Autodesk Fusion 360 part; units mm, degrees
note: some values were not read from the file. Chosen so that the rebuilt part matches the saved one: which face or edge a step refers to.
(part 2 of 2)
  line L527 (-26.0359, -3.6443) -> (-26.0026, -3.5739) construction
  line L528 (-26.0026, -3.5739) -> (-25.9789, -3.5255) construction
  line L529 (-25.9789, -3.5255) -> (-25.9665, -3.5003) construction
  line L530 (-121, -21.875) -> (-119, -21.875)
  line L531 (-119, -21.875) -> (-119, -56.875)
  line L532 (-119, -56.875) -> (-121, -56.875)
  line L533 (-60.5, -78.75) -> (-60.5, 0.0063) construction
  line L534 (-2, -56.875) -> (0, -56.875)
  line L535 (-2, -21.875) -> (-2, -56.875)
  line L536 (0, -21.875) -> (-2, -21.875)
  point P0 (0, -78.75)
  dimension "d4" = 5
  dimension "PlateWidthY" = 78.75
  dimension "d8" = 11.35
  dimension "OffsetY" = 6.725
  dimension "OffsetX" = 16.19
  dimension "PlateWidthX" = 117
  dimension "d21" = 6.875
  dimension "CapHolderWidth" = 13.4
  dimension "d27" = 2
  dimension "d28" = 2
  dimension "d29" = 2
  dimension "d38" = 2
  dimension "d39" = 80
  dimension "d47" = 2
  dimension "d48" = 2.5
  dimension "CapHolderAngle" = 45
  dimension "d50" = 2
  dimension "d51" = 35
  dimension "d52" = 17.5
  dimension "d53" = 10
  constraint horizontal L45
  constraint vertical L46
  constraint horizontal L47
  constraint vertical L48
  constraint coincident L54.start L53
  constraint perpendicular L49 L54
  constraint perpendicular L49 L50
  constraint parallel L49 L52
  constraint equal L51 L53
  constraint coincident L54 L53.end
  constraint coincident L50.start L51.start
  constraint coincident L46.start L56.start
  constraint coincident L45.end L56.end
  constraint coincident L55.end A0.centre
  constraint equal L50 L54
  constraint midpoint L49 L55.start
  constraint coincident origin L48
  constraint coincident L45 origin
  constraint tangent L48 A1
  constraint tangent L45 A1
  constraint coincident P0 L47
  constraint coincident P0 L48
  constraint tangent L47 A2
  constraint tangent L48 A2
  constraint tangent L46 A3
  constraint tangent L47 A3
  constraint perpendicular L47 L58
  constraint perpendicular L57 L59
  constraint equal L57 L58
  constraint perpendicular L58 L59
  constraint coincident L47 L57.start
  constraint midpoint L48 L60.start
  constraint coincident L46 L60.end
  constraint perpendicular L46 L60
  constraint symmetric L57.start L60 L62.start
  constraint symmetric L57.end L60 L61.end
  constraint symmetric L58.start L60 L61.start
  constraint symmetric L58.end L60 L63.end
  constraint perpendicular L52 L64
  constraint perpendicular L64 L65
  constraint perpendicular L65 L66
  constraint perpendicular L49 L55
  constraint coincident L48 L67.end
  constraint perpendicular L48 L67
  constraint coincident L46 L530.start
  constraint perpendicular L46 L530
  constraint coincident L46 L532.end
  constraint perpendicular L46 L532
  constraint perpendicular L531 L532
  constraint midpoint L47 L533.start
  constraint perpendicular L45 L533
  constraint symmetric L530.start L533 L536.start
  constraint symmetric L530.end L533 L535.start
  constraint symmetric L531.end L533 L534.start
  constraint symmetric L532.end L533 L534.end
  measures "d4" distance of L49 L52
  measures "PlateWidthY" distance of origin P0
  measures "d8" diameter of A0
  measures "OffsetY" distance of L45 L55.end
  measures "OffsetX" distance of L48 L55.end
  measures "PlateWidthX" distance of L45.end origin
  measures "d21" distance of L55.start L55.end
  measures "CapHolderWidth" distance of L49.start L49.end
  measures "d27" radius of A1
  measures "d28" radius of A2
  measures "d29" radius of A3
  measures "d38" distance of L58.start L58.end
  measures "d39" distance of L57.end L58.start
  measures "d47" distance of L52.end L64.end
  measures "d48" distance of L49.start L53.end
  measures "CapHolderAngle" angle of L55 L67
  measures "d50" distance of L530.start L530.end
  measures "d51" distance of L534.start L535.start
  measures "d52" distance of L60 L532
  measures "d53" distance of L64.end L65.end
extrude "Extrude1" add sketch "Sketch1" along normal blind 10 separate body contours L0 L1 L2 L3 L4 L5 L6 L7 | S0 L8 S1 S2 S3 L9 L10 L11 L12 L13 L14 S4 S5 L15 L17 L18 L19 L20 L21 L22 L23 L24 L25 L26 L27 L28 S6 S7 S8 S9 L29 L31 L32 L33 S10 S11 S12 S13 L34 S14 S15 S16 S17 L35 S18 L36 S19 S20 S21 S22 S23 S24 S25 L37 S26 S27 S28 L38 S29 S30 L45 L46 L47 L48 L56 A1 A2 A3 L57 L58 L59 L61 L62 L63 L530 L531 L532 L534 L535 L536 | S0 L8 S1 S2 S3 L9 L10 L11 L12 L13 L14 S4 S5 L61 | S1 S2 L15 L16 L17 L26 L27 L29 L30 L31 S20 S21 L45 L61 L62 L63 | S1 S2 L61 | S18 L36 S19 S20 S21 S22 S23 S24 S25 L37 S26 S27 S28 L38 S29 S30 L61 | S20 S21 L61 | L15 L17 L18 L19 L20 L21 L22 L23 L24 L25 L61 | L15 L16 L17 L61 | L26 L27 L61 | L26 L27 L28 S6 S7 S8 S9 L61 | L46 L530 L531 L532 | L29 L31 L32 L33 S10 S11 S12 S13 L34 S14 S15 S16 S17 L35 L61 | L29 L30 L31 L61 | L48 L534 L535 L536 | L47 L57 L58 L59 | L39 L40 L41 L42 L43 L44 | L49 L50 L51 L52 L53 L54 | L52 L64 L65 L66 | A0 makes body 2
extrude "Extrude2" cut sketch "Sketch1" along normal up to surface (10 mm away) contours L49 L50 L51 L52 L53 L54 | L52 L64 L65 L66 | A0 bodies 2
pattern_linear "R-Pattern1" count 6 spacing 18 along (-1, 0, 0) count 4 spacing 18 along (0, -1, 0) of "Extrude2"
extrude "Extrude3" cut sketch "Sketch1" along normal blind 1 contours S1 S2 L15 L16 L17 L26 L27 L29 L30 L31 S20 S21 L45 L61 L62 L63 | L26 L27 L61 | L46 L530 L531 L532 | L48 L534 L535 L536 | L47 L57 L58 L59 bodies 2
extrude "Extrude4" cut sketch "Sketch1" against normal blind 0.3 from surface at 10 contours L0 L1 L2 L3 L4 L5 L6 L7 | S0 L8 S1 S2 S3 L9 L10 L11 L12 L13 L14 S4 S5 L61 | S18 L36 S19 S20 S21 S22 S23 S24 S25 L37 S26 S27 S28 L38 S29 S30 L61 | L15 L17 L18 L19 L20 L21 L22 L23 L24 L25 L61 | L26 L27 L61 | L26 L27 L28 S6 S7 S8 S9 L61 | L29 L31 L32 L33 S10 S11 S12 S13 L34 S14 S15 S16 S17 L35 L61 | L39 L40 L41 L42 L43 L44 bodies 2
other "Modify1"
other "Modify2"
sketch "Sketch2" plane through (0, 0, 0) normal (0, 0, 1) x (1, 0, 0)
  circle A0 centre (-16.3744, -6.7737) radius 5.675
  circle A1 centre (-34.3633, -6.7765) radius 5.675
  dimension "d45" = 11.35
  dimension "d46" = 11.35
  measures "d45" diameter of A0
  measures "d46" diameter of A1
hidden bodies 1
equation "CapHolderBevelAngle = 135.00 deg"
equation "PlateDepth = 10 mm"
equation "Count = 24 mm"
equation "CountX = ( ( if(Count == 12 mm; 4; if(Count == 24 mm; 6; if(Count == 48 mm; 8; if(Count == 96 mm; 12; 1)))) ) * 1 ) * 1 mm"
equation "CountY = ( Count / CountX ) * 1 mm"
equation "Spacing = ( if(Count == 12 mm; 26; if(Count == 24 mm; 18; if(Count == 48 mm; 13; if(Count == 96 mm; 9; 1)))) ) * 1 mm"
equation "d30 = PlateDepth"
equation "CountX1 = ( ( if(Count == 12 mm; 4; if(Count == 24 mm; 6; if(Count == 48 mm; 8; if(Count == 96 mm; 12; 1)))) ) * 1 ) * 1"
equation "CountY1 = ( Count / CountX )"
equation "d36 = Spacing"
equation "d37 = -Spacing"
